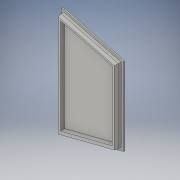
# Autodesk Inventor part: FoodHopperLid
Saved by Autodesk Inventor 2016 (Build 200138000, 138)
## iProperties
Created: 2016-04-07
Part Number: FoodHopperLid
Material: Generic
Document SubType Name: Modeling
Designer: reinert
Density: 1 g/cm^3
Appearance: Default
Author: reinert
Autodesk Inventor part; units mm, degrees
ref_plane "YZ Plane" through (0, 0, 0) normal (1, 0, 0) x (0, 1, 0)
ref_plane "XZ Plane" through (0, 0, 0) normal (0, 1, 0) x (-1, 0, 0)
ref_plane "XY Plane" through (0, 0, 0) normal (0, 0, 1) x (1, 0, 0)
sketch "Sketch1" plane through (0, 0, 0) normal (0, 1, 0) x (-1, 0, 0)
  line L0 (0, 0) -> (0, -109)
  line L1 (0, -109) -> (84.3015, -130.5)
  line L2 (84.3015, -130.5) -> (84.3015, 21.5)
  line L3 (0, 0) -> (84.3015, 21.5)
  dimension "d0" = 109
  dimension "d3" = 87
  dimension "d4" = 152
  dimension "d5" = 87
  constraints: 8 end point, 1 parallel, 1 vertical
  measures "d0" distance of L0.start L0.end
  measures "d3" distance of L0.end L1.end
  measures "d4" distance of L1.end L2.end
  measures "d5" distance of L2.end L0.start
extrude "Extrusion1" add sketch "Sketch1" along normal blind 4
sketch "Sketch2" plane through (0, 0, 0) normal (0, -1, 0) x (1, 0, 0)
  line L0 (0, 0) -> (0, -109) projected
  line L1 (0, -109) -> (-5, -109)
  line L2 (-4.8329, -103.795) -> (-4.8329, -3.205)
  line L3 (-5, 0) -> (0, 0)
  line L4 (0, 0) -> (0, -109)
  line L5 (0, -109) -> (-84.3015, -130.5) projected
  line L6 (-84.3015, -130.5) -> (-74.4446, -130.5)
  line L7 (-79.3015, 21.5) -> (-84.3015, 21.5)
  line L8 (-84.3015, 21.5) -> (-84.3015, -130.5)
  line L9 (-84.3015, -130.5) -> (0, -109)
  line L10 (0, -109) -> (-1.2356, -104.1551)
  line L11 (-85.5402, -125.6434) -> (-84.3015, -130.5)
  line L12 (-84.3015, -130.5) -> (-84.3015, 21.5) projected
  line L13 (0, 0) -> (-84.3015, 21.5)
  line L14 (-84.3015, 21.5) -> (-85.5372, 16.6551)
  line L15 (-1.4353, -5.628) -> (0, 0)
  line L16 (-74.4446, -130.5) -> (-74.4446, -127.9861)
  line L17 (-4.8329, -103.795) -> (-74.2654, -121.5028)
  line L18 (-84.3015, -125.3275) -> (-85.5402, -125.6434)
  line L19 (-85.5372, 16.6551) -> (-84.3015, 16.34)
  line L20 (-74.2654, 14.5028) -> (-4.8329, -3.205)
  line L21 (-79.3015, 20.2248) -> (-79.3015, 21.5)
  line L22 (-79.3015, 15.8371) -> (-79.3015, -122.7872)
  line L23 (-74.2654, -121.5028) -> (-79.3015, -122.7872)
  line L24 (-74.2654, 14.5028) -> (-79.3015, 15.8371)
  dimension "d9" = 5
  dimension "d10" = 5
  dimension "d11" = 5
  dimension "d12" = 5
  constraints: 44 end point, 12 parallel, 6 perpendicular, 4 point on line, 2 horizontal, 1 collinear
  measures "d9" distance of L0.start L3.start
  measures "d10" distance of L7.end L7.start
  measures "d11" distance of L10.end L0.end
  measures "d12" distance of L14.end L7.end
extrude "Extrusion2" add sketch "Sketch2" along normal blind 5 draft -10 contours L0 L5 L8 L13
sketch "Sketch3" plane through (0, 4, 0) normal (0, 1, 0) x (1, 0, 0)
  line L0 (0, 34.4959) -> (3, 34.4959) construction
  line L1 (3.8363, -2.2322) -> (3.8363, 112.6381)
  line L2 (-79.382, 43.4403) -> (-76.382, 43.4403) construction
  line L3 (-84.3015, 130.5) -> (-84.3015, -21.5) projected
  line L4 (-84.3015, 135.1165) -> (3.8363, 112.6381)
  line L5 (0, 109) -> (-84.3015, 130.5) projected
  line L6 (3.8363, -2.2322) -> (-84.3015, -24.7106)
  line L7 (-84.3015, -21.5) -> (0, 0) projected
  line L8 (-84.3015, 130.5) -> (-84.3015, 135.1165)
  line L9 (-84.3015, -21.5) -> (-84.3015, -24.7106)
  line L10 (-84.3015, 135.1165) -> (-88.3015, 135.1165)
  line L11 (-88.3015, 135.1165) -> (-88.3015, -24.7106)
  line L12 (-88.3015, -24.7106) -> (-84.3015, -24.7106)
  line L13 (-84.3015, -24.7106) -> (-84.3015, 135.1165)
  dimension "d24" = 4
  constraints: 22 end point, 4 parallel, 3 horizontal, 3 vertical, 1 perpendicular
  measures "d24" distance of L12.end L11.end
extrude "Extrusion3" add sketch "Sketch3" along normal blind 2
body "Solid1"
